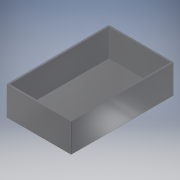
# Autodesk Inventor part: Batterybox
Saved by Autodesk Inventor 2018 (Build 220112000, 112)
## iProperties
Created: 2018-08-07
Part Number: Batterybox
Material: Generic
Document SubType Name: Modeling
Designer: ruben
Density: 1 g/cm^3
Sheet Metal Rule: Default_mm
Appearance: Aluminum - Dark
Author: ruben
Autodesk Inventor part; units mm, degrees
ref_plane "YZ Plane" through (0, 0, 0) normal (1, 0, 0) x (0, 1, 0)
ref_plane "XZ Plane" through (0, 0, 0) normal (0, 1, 0) x (-1, 0, 0)
ref_plane "XY Plane" through (0, 0, 0) normal (0, 0, 1) x (1, 0, 0)
sketch "Sketch3" plane through (0, 0, 0) normal (0, 0, 1) x (1, 0, 0)
  line L0 (0, -133) -> (0, 133) projected
  line L1 (-210, 0) -> (210, 0) projected
  line L2 (-150, -95) -> (150, -95)
  line L3 (150, -95) -> (150, 95)
  line L4 (150, 95) -> (-150, 95)
  line L5 (-150, 95) -> (-150, -95)
  line L6 (-150, -95) -> (150, 95) construction
  line L7 (150, -95) -> (-150, 95) construction
  line L8 (-145, -90) -> (145, -90)
  line L9 (145, -90) -> (145, 90)
  line L10 (145, 90) -> (-145, 90)
  line L11 (-145, 90) -> (-145, -90)
  line L12 (-145, -90) -> (145, 90) construction
  line L13 (145, -90) -> (-145, 90) construction
  point P0 (0, 0)
  dimension "d0" = 300
  dimension "d1" = 190
  dimension "d2" = 290
  dimension "d3" = 180
  constraints: 24 end point, 4 midpoint, 4 parallel, 2 horizontal, 2 perpendicular
  measures "d0" distance of L4.end L3.end
  measures "d1" distance of L3.end L2.end
  measures "d2" distance of L9.end L10.end
  measures "d3" distance of L8.end L9.end
extrude "Extrusion1" add sketch "Sketch3" along normal blind 85 contours L2 L5 L1 L11 L8 L0 | L0 L8 L9 L1 L3 L2 | L5 L4 L0 L10 L11 L1 | L1 L9 L10 L0 L4 L3
extrude "Extrusion2" add sketch "Sketch3" along normal blind 5 contours L8 L11 L1 L0 | L0 L1 L9 L8 | L1 L11 L10 L0 | L0 L10 L9 L1
fillet "Fillet1" radius 2 8 edges at (150, -95, 42.5) (150, 95, 42.5) (-150, 95, 42.5) (-150, -95, 42.5) (-150, 0, 0) (0, 95, 0) (0, -95, 0) (150, 0, 0)
equation "\"BendRadius\" = Thickness"
equation "\"BendReliefWidth\" = Thickness"
equation "\"BendReliefDepth\" = 0.5 * Thickness"
equation "\"CornerReliefSize\" = 4 * Thickness"
equation "\"MinimumRemnant\" = 2 * Thickness"
equation "\"TransitionRadius\" = BendRadius"
equation "\"JacobiRadiusSize\" = BendRadius"
equation "\"GapSize\" = Thickness"
equation "\"Thickness\" = 0.5"
body "Solid1"
